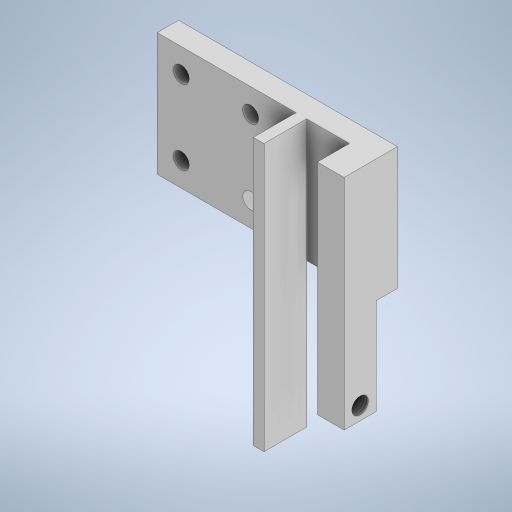
# Autodesk Inventor part: робот-энкодер
Saved by Autodesk Inventor 2024.2 (Build 282272000, 272)
## iProperties
Created: 2025-11-27
Part Number: робот-энкодер
Material: Типовые
Document SubType Name: Modeling
Designer: Zakhar
Density: 1 g/cm^3
Appearance: По умолчанию
Author: Zakhar
Autodesk Inventor part; units mm, degrees
ref_plane "YZ Plane" through (0, 0, 0) normal (1, 0, 0) x (0, 1, 0)
ref_plane "XZ Plane" through (0, 0, 0) normal (0, 1, 0) x (-1, 0, 0)
ref_plane "XY Plane" through (0, 0, 0) normal (0, 0, 1) x (1, 0, 0)
ref_plane "РабПлоскость1" through (0, 0, 0) normal (0, 0, 1) x (1, 0, 0)
sketch "Эскиз1" plane through (0, 0, 0) normal (0, 0, 1) x (1, 0, 0)
  circle A0 centre (22, -74) radius 1.5
  circle A1 centre (22, -60) radius 1.5
  circle A2 centre (35, -74) radius 1.5
  circle A3 centre (35, -60) radius 1.5
  line L0 (26, -96) -> (10, -96) projected
  line L1 (32, -92) -> (10, -92) projected
  line L2 (48, -70) -> (48, -50) projected
  line L3 (48, -90) -> (48, -70) projected
  line L4 (17.5, -78.5) -> (58.5, -78.5)
  line L5 (58.5, -78.5) -> (58.5, -55.5)
  line L6 (58.5, -55.5) -> (17.5, -55.5)
  line L7 (17.5, -55.5) -> (17.5, -78.5)
  point P0 (0, 0)
  point P1 (21, -92)
  dimension "d0" = 18
  dimension "d1" = 18
  dimension "d2" = 14
  dimension "d3" = 14
  dimension "d4" = 3
  dimension "d5" = 3
  dimension "d6" = 3
  dimension "d7" = 3
  dimension "d8" = 13
  dimension "d9" = 13
  dimension "d10" = 13
  dimension "d11" = 13
  dimension "d12" = 23
  dimension "d13" = 41
  dimension "d14" = 4.5
  dimension "d15" = 4.5
  constraints: 8 end point, 4 centre point, 2 parallel, 1 horizontal, 1 midpoint, 1 perpendicular
  measures "d0" vertical distance of point (21, -92) A0.centre
  measures "d1" distance from line of L1 A2.centre
  measures "d2" distance of A0.centre A1.centre
  measures "d3" distance of A2.centre A3.centre
  measures "d4" diameter of A3
  measures "d5" diameter of A1
  measures "d6" diameter of A0
  measures "d7" diameter of A2
  measures "d8" distance from line of A2.centre L3
  measures "d9" distance of A2.centre A0.centre
  measures "d10" distance from line of L2 A3.centre
  measures "d11" distance of A3.centre A1.centre
  measures "d12" distance of L4.end L5.end
  measures "d13" distance of L5.end L6.end
  measures "d14" distance from line of L7 A0.centre
  measures "d15" distance from line of L4 A0.centre
extrude "Выдавливание1" add sketch "Эскиз1" along normal blind 4
sketch "Эскиз2" plane through (0, 0, 4) normal (0, 0, 1) x (1, 0, 0)
  line L0 (43.5, -105.5) -> (45.5, -105.5)
  line L1 (45.5, -105.5) -> (45.5, -55.5)
  line L2 (45.5, -55.5) -> (43.5, -55.5)
  line L3 (43.5, -55.5) -> (43.5, -105.5)
  line L4 (53.5, -55.5) -> (58.5, -55.5)
  line L5 (58.5, -55.5) -> (58.5, -96.5)
  line L6 (58.5, -96.5) -> (53.5, -96.5)
  line L7 (53.5, -96.5) -> (53.5, -55.5)
  line L8 (58.5, -78.5) -> (58.5, -55.5) projected
  line L9 (58.5, -55.5) -> (17.5, -55.5) projected
  line L10 (17.5, -78.5) -> (58.5, -78.5) projected
  point P0 (0, 0)
  point P1 (53.5, -78.5)
  dimension "d18" = 8
  dimension "d19" = 18
  dimension "d20" = 5
  dimension "d21" = 2
  dimension "d22" = 50
  constraints: 16 end point, 4 parallel, 3 collinear, 2 horizontal, 2 perpendicular
  measures "d18" distance between parallel lines of L1 L7
  measures "d19" distance between parallel lines of L10 L6
  measures "d20" distance between parallel lines of L5 L7
  measures "d21" distance between parallel lines of L1 L3
  measures "d22" distance of L2.end L0.start
extrude "Выдавливание2" add sketch "Эскиз2" along normal blind 6 contours L10 L5 L6 L7 | L7 L4 L5 L10
sketch "Эскиз3" plane through (53.5, -96.5, 4) normal (-1, 0, 0) x (0, 0, 1)
  line L0 (6, 41) -> (6, -9) projected
  line L1 (0, 18) -> (0, 41) projected
  line L2 (0, 18) -> (0, -9) projected
  line L3 (0, -9) -> (6, -9) projected
  line L4 (6, 41) -> (6, -9) projected
  line L5 (0, 41) -> (6, 41) projected
  circle A0 centre (3, 2.5) radius 1.55
  line L6 (-4, 18) -> (0, 18) projected
  point P0 (-4, 96.5)
  dimension "d25" = 15.5
  dimension "d26" = 3.1
  constraints: 1 centre point
  measures "d25" distance from line of L6 A0.centre
  measures "d26" diameter of A0
extrude "Выдавливание3" cut sketch "Эскиз3" against normal through all contours A0
thread "Резьба1" size "M3x0.5" class "6H" standard "ANSI Metric M Profile" full length
extrude "Выдавливание4" add sketch "Эскиз2" along normal blind 8 contours L3 L10 L1 L0 | L3 L2 L1 L10
